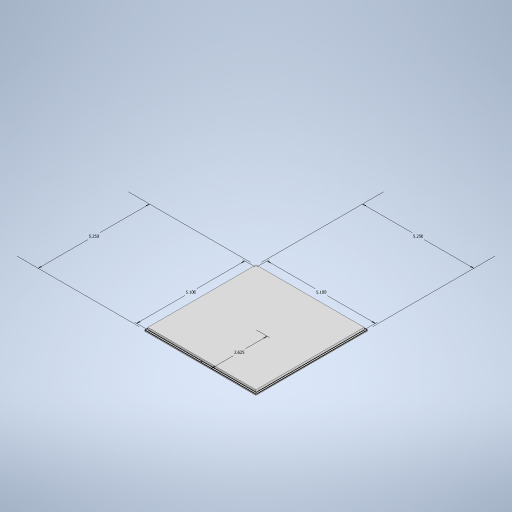
# Autodesk Inventor part: TC720 lid
Saved by Autodesk Inventor 2024.1 (Build 281209000, 209)
## iProperties
Created: 2024-09-06
Part Number: TC720 lid
Material: Generic
Document SubType Name: Modeling
Designer: pab2
Density: 1 g/cm^3
Appearance: Default
Author: pab2
Autodesk Inventor part; units mm, degrees
ref_plane "YZ Plane" through (0, 0, 0) normal (1, 0, 0) x (0, 1, 0)
ref_plane "XZ Plane" through (0, 0, 0) normal (0, 1, 0) x (-1, 0, 0)
ref_plane "XY Plane" through (0, 0, 0) normal (0, 0, 1) x (1, 0, 0)
sketch "Sketch1" plane through (0, 0, 0) normal (0, 1, 0) x (-1, 0, 0)
  line L0 (0, 0) -> (133.35, 0)
  line L1 (133.35, 0) -> (133.35, -133.35)
  line L2 (133.35, -133.35) -> (0, -133.35)
  line L3 (0, -133.35) -> (0, 0)
  line L4 (66.675, 0) -> (66.675, -66.675)
  line L5 (1.905, -1.905) -> (131.445, -1.905)
  line L6 (131.445, -1.905) -> (131.445, -131.445)
  line L7 (131.445, -131.445) -> (1.905, -131.445)
  line L8 (1.905, -131.445) -> (1.905, -1.905)
  line L9 (1.905, -1.905) -> (131.445, -131.445) construction
  line L10 (131.445, -1.905) -> (1.905, -131.445) construction
  dimension "d0" = 133.35
  dimension "d1" = 133.35
  dimension "d2" = 66.675
  dimension "d3" = 129.54
  dimension "d4" = 129.54
  constraints: 22 end point, 4 parallel, 3 midpoint, 2 horizontal, 2 perpendicular, 1 vertical
  measures "d0" distance of L1.end L2.end
  measures "d1" distance of L0.end L1.end
  measures "d2" distance of L4.start L4.end
  measures "d3" distance of L6.end L7.end
  measures "d4" distance of L5.end L6.end
extrude "Extrusion1" add sketch "Sketch1" along normal blind 2.54 contours L5 L6 L7 L8
extrude "Extrusion2" add sketch "Sketch1" against normal blind 2.54 contours L5 L6 L7 L8 | L0 L1 L2 L3
fillet "Fillet1" radius 1.27 4 edges at (-133.35, -2.54, -66.675) (-66.675, -2.54, -133.35) (-66.675, -2.54, 0) (0, -2.54, -66.675)
body "Solid1"
